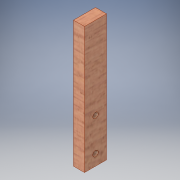
# Autodesk Inventor part: Sensor_Halterung_Teil1
Saved by Autodesk Inventor 2018 (Build 220112000, 112)
## iProperties
Created: 2018-03-26
Part Number: Sensor_Halterung_Teil1
Material: Holz (Eiche)
Document SubType Name: Modeling
Designer: Julian
Density: 0.76 g/cm^3
Appearance: Weißeiche - natur - mittlerer Glanz
Author: Julian
Autodesk Inventor part; units mm, degrees
ref_plane "YZ Plane" through (0, 0, 0) normal (1, 0, 0) x (0, 1, 0)
ref_plane "XZ Plane" through (0, 0, 0) normal (0, 1, 0) x (-1, 0, 0)
ref_plane "XY Plane" through (0, 0, 0) normal (0, 0, 1) x (1, 0, 0)
sketch "Skizze1" plane through (0, 0, 0) normal (0, 1, 0) x (-1, 0, 0)
  line L0 (0, 0) -> (10, 0)
  line L1 (10, 0) -> (10, -115)
  line L2 (10, -115) -> (0, -115)
  line L3 (0, -115) -> (0, 0)
  dimension "d0" = 10
  dimension "d1" = 115
  constraints: 8 end point, 2 parallel, 1 horizontal, 1 perpendicular
  measures "d0" distance of L1.end L2.end
  measures "d1" distance of L0.end L1.end
extrude "Extrusion1" add sketch "Skizze1" along normal blind 20
sketch "Skizze2" plane through (0, 20, 0) normal (0, 1, 0) x (1, 0, 0)
  line L0 (0, 0) -> (-5, 0)
  line L1 (-10, 0) -> (0, 0) projected
  line L2 (-5, 0) -> (-5, 2.25)
  line L3 (-5, 2.25) -> (-5, 17.75)
  dimension "d4" = 2.25
  dimension "d5" = 15.5
  constraints: 6 end point, 1 midpoint, 1 perpendicular, 1 point on line
  measures "d4" distance of L0.end L2.end
  measures "d5" distance of L2.end L3.end
hole "Bohrung1" at (-5, 20, -2.25) at (-5, 20, -17.75) direction (0, -1, 0) diameter 2.5 depth 8 tip angle 118
sketch "Skizze3" plane through (0, 0, 0) normal (1, 0, 0) x (0, 0, -1)
  line L0 (115, 0) -> (0, 0) projected
  line L1 (115, 0) -> (115, 10)
  line L2 (115, 0) -> (115, 20) projected
  line L3 (115, 10) -> (65, 10)
  line L4 (65, 10) -> (75, 10)
  line L5 (75, 10) -> (105, 10)
  dimension "d13" = 50
  dimension "d14" = 10
  dimension "d15" = 30
  constraints: 8 end point, 2 point on line, 1 midpoint, 1 perpendicular
  measures "d13" distance of L1.end L3.end
  measures "d14" distance of L3.end L4.end
  measures "d15" distance of L4.end L5.end
hole "Bohrung2" at (0, 10, -75) at (0, 10, -105) direction (-1, 0, 0) diameter 5 end through all
